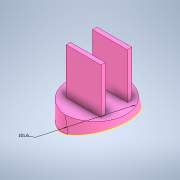
# Autodesk Inventor part: bracketForGarageUpperHalfV02
Saved by Autodesk Inventor 2022.2 (Build 262287000, 287)
## iProperties
Created: 2021-10-20
Part Number: bracketForGarageUpperHalfV02
Material: PC/ABS Plastic
Document SubType Name: Modeling
Designer: robst
Density: 0.357273 g/cm^3
Appearance: Pink
Author: robst
Autodesk Inventor part; units mm, degrees
ref_plane "YZ Plane" through (0, 0, 0) normal (1, 0, 0) x (0, 1, 0)
ref_plane "XZ Plane" through (0, 0, 0) normal (0, 1, 0) x (-1, 0, 0)
ref_plane "XY Plane" through (0, 0, 0) normal (0, 0, 1) x (1, 0, 0)
sketch "Sketch50" plane through (0, 0, 0) normal (0, 1, 0) x (-1, 0, 0)
  circle A0 centre (0, 0) radius 57.15
  dimension "d230" = 114.3
  constraints: 1 centre point, 1 coincident
  measures "d230" diameter of A0
extrude "Extrusion25" add sketch "Sketch50" against normal blind 8
sketch "Sketch51" plane through (0, 0, 0) normal (0, 1, 0) x (1, 0, 0)
  line L0 (-32.229, -20.32) -> (32.229, -20.32)
  line L1 (-32.229, 20.32) -> (32.229, 20.32)
  line L2 (-25.487, -28.32) -> (25.487, -28.32)
  line L3 (-25.487, 28.32) -> (25.487, 28.32)
  line L4 (-32.229, -20.32) -> (-32.229, -28.32)
  line L5 (-32.229, -28.32) -> (-25.487, -28.32)
  line L6 (32.229, -20.32) -> (32.229, -28.32)
  line L7 (32.229, -28.32) -> (25.487, -28.32)
  line L8 (-32.229, 20.32) -> (-32.229, 28.32)
  line L9 (-32.229, 28.32) -> (-25.487, 28.32)
  line L10 (32.229, 20.32) -> (32.229, 28.32)
  line L11 (25.487, 28.32) -> (32.229, 28.32)
  point P0 (0, 0)
  dimension "d234" = 40.64
  dimension "d235" = 8
  constraints: 24 end point, 6 perpendicular, 5 parallel, 4 point on line, 1 horizontal, 1 vertical
  measures "d234" distance between parallel lines of L1 L0
  measures "d235" distance between parallel lines of L0 L2
extrude "Extrusion26" add sketch "Sketch51" along normal blind 84.1375
sketch "Sketch54" plane through (0, 0, 0) normal (0, 0, 1) x (1, 0, 0)
  line L0 (-57.15, -8) -> (57.15, -8) projected
  line L1 (57.15, -8) -> (-57.15, -49.6018)
  line L2 (-57.15, -49.6018) -> (-57.15, -8)
  line L3 (57.15, 0) -> (-57.15, 0) projected
  point P0 (0, 0)
  dimension "d249" = 20
  constraints: 4 end point, 1 perpendicular
  measures "d249" angle of L1 L0
extrude "Extrusion28" add sketch "Sketch54" along normal up to surface round surface about axis through (0, 0, 0) along (0, -1, 0) radius 57.15 far side no
mirror "Mirror3" about plane through (0, 0, 0) normal (0, 0, 1) of "Extrusion28"
sketch "Sketch55" plane through (0, -28.8009, 0) normal (0.3420201, -0.9396926, 0) x (0.9396926, 0.3420201, 0)
  circle A0 centre (0, 0) radius 57.15
  circle A1 centre (0, 0) radius 69.85
  point P0 (9.8505, 0)
  dimension "d252" = 114.3
  dimension "d255" = 139.7
  constraints: 2 centre point, 2 coincident
  measures "d252" diameter of A0
  measures "d255" diameter of A1
extrude "Extrusion30" cut sketch "Sketch55" against normal blind 30.649
sketch "Sketch56" plane through (0, -28.8009, 0) normal (0.3420201, -0.9396926, 0) x (0.9396926, 0.3420201, 0)
  arc A0 (0, 57.15) -> (0, -57.15) centre (0, 0) ccw projected
  arc A1 (0, -57.15) -> (0, 57.15) centre (0, 0) ccw projected
  circle A2 centre (0, 0) radius 50.8 construction
  point P0 (9.8505, 0)
  point P1 (-50.8, 0)
  dimension "d258" = 101.6
  constraints: 1 coincident, 1 horizontal alignment, 2 other
equation "\"d230\" = outsideDiameter"
equation "\"d231\" = wallThickness"
equation "\"d234\" = twoByFourWidth"
equation "\"d235\" = wallThickness"
equation "\"d236\" = twoByFourDepth"
equation "\"wallThickness\" = 8"
equation "\"twoByFourWidth\" = 40.64"
equation "\"twoByFourDepth\" = 84.1375"
equation "\"azimuth\" = -15deg"
equation "\"elevation\" = 20deg"
equation "\"centerForTwoHoles\" = 0.25 * diagonalLine"
equation "\"depthOfExtrusionForMatingToLowerHalf\" = 12.5"
equation "\"depthForWasherForMatingToCase\" = 14"
equation "\"outsideDiameter\" = 114.3"
equation "\"diagonalLine\" = 85.134222"
body "Solid4"
